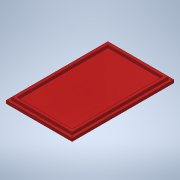
# Autodesk Inventor part: Enclose Bottom
Saved by Autodesk Inventor 2022.3 (Build 263350030, 350C)
## iProperties
Created: 2025-03-25
Part Number: Enclose Bottom
Material: PC/ABS Plastic
Document SubType Name: Modeling
Designer: EJErickson
Density: 0.357273 g/cm^3
Appearance: Light Red
Author: EJErickson
Autodesk Inventor part; units mm, degrees
ref_plane "YZ Plane" through (0, 0, 0) normal (1, 0, 0) x (0, 1, 0)
ref_plane "XZ Plane" through (0, 0, 0) normal (0, 1, 0) x (-1, 0, 0)
ref_plane "XY Plane" through (0, 0, 0) normal (0, 0, 1) x (1, 0, 0)
sketch "Sketch1" plane through (0, 0, 0) normal (0, 1, 0) x (-1, 0, 0)
  line L0 (-60, 92.5) -> (60, 92.5)
  line L1 (60, 92.5) -> (60, -92.5)
  line L2 (60, -92.5) -> (-60, -92.5)
  line L3 (-60, -92.5) -> (-60, 92.5)
  line L4 (-60, 92.5) -> (60, -92.5) construction
  line L5 (60, 92.5) -> (-60, -92.5) construction
  point P0 (0, 0)
  dimension "d0" = 120
  dimension "d1" = 185
  constraints: 12 end point, 2 midpoint, 2 parallel, 1 horizontal, 1 perpendicular
  measures "d0" distance of L1.end L2.end
  measures "d1" distance of L0.end L1.end
extrude "Extrusion1" add sketch "Sketch1" along normal blind 5
sketch "Sketch2" plane through (0, 5, 0) normal (0, 1, 0) x (1, 0, 0)
  line L0 (55, -87.5) -> (-55, -87.5)
  line L1 (-55, -87.5) -> (-55, 87.5)
  line L2 (-55, 87.5) -> (55, 87.5)
  line L3 (55, 87.5) -> (55, -87.5)
  line L4 (55, -87.5) -> (-55, 87.5) construction
  line L5 (-55, -87.5) -> (55, 87.5) construction
  line L6 (50, -82.5) -> (-50, -82.5)
  line L7 (-50, -82.5) -> (-50, 82.5)
  line L8 (-50, 82.5) -> (50, 82.5)
  line L9 (50, 82.5) -> (50, -82.5)
  line L10 (50, -82.5) -> (-50, 82.5) construction
  line L11 (-50, -82.5) -> (50, 82.5) construction
  point P0 (0, 0)
  dimension "d4" = 110
  dimension "d5" = 175
  dimension "d6" = 100
  dimension "d7" = 165
  constraints: 24 end point, 4 midpoint, 4 parallel, 2 horizontal, 2 perpendicular
  measures "d4" distance of L1.end L2.end
  measures "d5" distance of L0.end L1.end
  measures "d6" distance of L7.end L8.end
  measures "d7" distance of L6.end L7.end
extrude "Extrusion2" add sketch "Sketch2" along normal blind 5
sketch "Sketch4" plane through (0, 5, 0) normal (0, 1, 0) x (1, 0, 0)
  circle A0 centre (57.5, -90) radius 1.625
  circle A1 centre (57.5, 90) radius 1.625
  circle A2 centre (-57.5, 90) radius 1.625
  circle A3 centre (-57.5, -90) radius 1.625
  point P0 (0, 0)
  dimension "d11" = 3.25
  dimension "d12" = 3.25
  dimension "d13" = 3.25
  dimension "d16" = 3.25
  constraints: 4 centre point
  measures "d11" diameter of A0
  measures "d12" diameter of A1
  measures "d13" diameter of A2
  measures "d16" diameter of A3
extrude "Extrusion3" cut sketch "Sketch4" against normal blind 5
sketch "Sketch5" plane through (0, 5, 0) normal (0, 1, 0) x (1, 0, 0)
  circle A0 centre (57.5, 90) radius 1.625 projected
  circle A1 centre (57.5, 90) radius 1.625
  circle A2 centre (57.5, -90) radius 1.625 projected
  circle A3 centre (57.5, -90) radius 1.625
  circle A4 centre (-57.5, -90) radius 1.625 projected
  circle A5 centre (-57.5, -90) radius 1.625
  circle A6 centre (-57.5, 90) radius 1.625 projected
  circle A7 centre (-57.5, 90) radius 1.625
  point P0 (0, 0)
  constraints: 4 centre point, 4 coincident
extrude "Extrusion4" add sketch "Sketch5" against normal blind 2
sketch "Sketch6" plane through (0, 5, 0) normal (0, 1, 0) x (1, 0, 0)
  circle A0 centre (57.5, 90) radius 1.625 projected
  circle A1 centre (57.5, 90) radius 0.75
  circle A2 centre (57.5, -90) radius 1.625 projected
  circle A3 centre (57.5, -90) radius 0.75
  circle A4 centre (-57.5, -90) radius 1.625 projected
  circle A5 centre (-57.5, -90) radius 0.75
  circle A6 centre (-57.5, 90) radius 1.625 projected
  circle A7 centre (-57.5, 90) radius 0.75
  point P0 (0, 0)
  dimension "d19" = 1.5
  dimension "d20" = 1.5
  dimension "d21" = 1.5
  dimension "d22" = 1.5
  constraints: 4 centre point, 4 coincident
  measures "d19" diameter of A1
  measures "d20" diameter of A3
  measures "d21" diameter of A5
  measures "d22" diameter of A7
extrude "Extrusion5" cut sketch "Sketch6" against normal blind 2 contours A1 | A3 | A5 | A7
body "Solid1"
